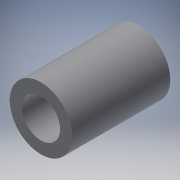
# Autodesk Inventor part: newRollerBearing
Saved by Autodesk Inventor 2019 (Build 230136000, 136)
## iProperties
Created: 2021-11-20
Part Number: newRollerBearing
Material: Generic
Document SubType Name: Modeling
Designer: Ian
Density: 1 g/cm^3
Appearance: Default
Author: Ian
Autodesk Inventor part; units mm, degrees
ref_plane "YZ Plane" through (0, 0, 0) normal (1, 0, 0) x (0, 1, 0)
ref_plane "XZ Plane" through (0, 0, 0) normal (0, 1, 0) x (-1, 0, 0)
ref_plane "XY Plane" through (0, 0, 0) normal (0, 0, 1) x (1, 0, 0)
sketch "Sketch1" plane through (0, 0, 0) normal (0, 0, 1) x (1, 0, 0)
  circle A0 centre (0, -1.9394) radius 2 construction
  circle A1 centre (0, -1.9394) radius 2.15
  circle A2 centre (0, -1.9394) radius 4
  point P0 (0, 0)
  dimension "d0" = 4
  dimension "d1" = 0.15
  dimension "d2" = 8
  constraints: 2 centre point, 1 coincident
  measures "d0" diameter of A0
  measures "d1" radial gap between concentric circles of A0 A1
  measures "d2" diameter of A2
extrude "Extrusion1" add sketch "Sketch1" along normal blind 11
sketch "Sketch2" plane through (0, 0, 0) normal (1, 0, 0) x (0, 1, 0)
  line L0 (2.0606, 0) -> (2.0606, 11) construction
  line L1 (-11.0374, 8.4) -> (-11.0374, 8.56) construction
  line L2 (-11.6374, 9.04) -> (-11.6374, 8.88) construction
  line L3 (-11.0374, 9.36) -> (-11.6374, 9.04) construction
  line L4 (-11.6374, 8.88) -> (-11.0374, 8.56) construction
  line L5 (-11.0374, 8.4) -> (-11.6374, 8.08) construction
  line L6 (-11.6374, 8.08) -> (-11.6374, 7.92) construction
  line L7 (-11.6374, 7.92) -> (-11.0374, 7.6) construction
  line L8 (-11.6374, 8.88) -> (2.0606, 8.88) construction
  line L9 (2.0606, 8.88) -> (1.4606, 8.56)
  line L10 (1.4606, 8.56) -> (1.4606, 8.4)
  line L11 (1.4606, 8.4) -> (2.0606, 8.08)
  line L12 (2.0606, 8.08) -> (2.0606, 7.92)
  line L13 (2.0606, 7.12) -> (2.0606, 6.96)
  line L14 (1.4606, 7.44) -> (2.0606, 7.12)
  line L15 (1.4606, 7.6) -> (1.4606, 7.44)
  line L16 (2.0606, 7.92) -> (1.4606, 7.6)
  line L17 (2.0606, 6.16) -> (2.0606, 6)
  line L18 (1.4606, 6.48) -> (2.0606, 6.16)
  line L19 (1.4606, 6.64) -> (1.4606, 6.48)
  line L20 (2.0606, 6.96) -> (1.4606, 6.64)
  line L21 (2.0606, 5.2) -> (2.0606, 5.04)
  line L22 (1.4606, 5.52) -> (2.0606, 5.2)
  line L23 (1.4606, 5.68) -> (1.4606, 5.52)
  line L24 (2.0606, 6) -> (1.4606, 5.68)
  line L25 (2.0606, 4.24) -> (2.0606, 4.08)
  line L26 (1.4606, 4.56) -> (2.0606, 4.24)
  line L27 (1.4606, 4.72) -> (1.4606, 4.56)
  line L28 (2.0606, 5.04) -> (1.4606, 4.72)
  line L29 (2.0606, 3.28) -> (2.0606, 3.12)
  line L30 (1.4606, 3.6) -> (2.0606, 3.28)
  line L31 (1.4606, 3.76) -> (1.4606, 3.6)
  line L32 (2.0606, 4.08) -> (1.4606, 3.76)
  line L33 (2.0606, 2.32) -> (2.0606, 2.16)
  line L34 (1.4606, 2.64) -> (2.0606, 2.32)
  line L35 (1.4606, 2.8) -> (1.4606, 2.64)
  line L36 (2.0606, 3.12) -> (1.4606, 2.8)
  line L37 (2.0606, 8.88) -> (2.0606, 8.08)
  line L38 (2.0606, 7.92) -> (2.0606, 7.12)
  line L39 (2.0606, 6.96) -> (2.0606, 6.16)
  line L40 (2.0606, 6) -> (2.0606, 5.2)
  line L41 (2.0606, 5.04) -> (2.0606, 4.24)
  line L42 (2.0606, 4.08) -> (2.0606, 3.28)
  line L43 (2.0606, 3.12) -> (2.0606, 2.32)
  line L44 (-1.9394, 10.1386) -> (-1.9394, 4.0681) construction
  line L45 (0.2106, 0) -> (0.2106, 11) construction
  line L46 (-4.0894, 0) -> (-4.0894, 11) construction
  point P0 (0, 0)
  dimension "d5" = 0.16
  dimension "d6" = 0.16
  dimension "d7" = 0.8
  dimension "d8" = 0.6
  dimension "d9" = 0.6
  dimension "d10" = 0.8
  dimension "d13" = 0.96
  dimension "d18" = 2.15
  dimension "d19" = 2.15
  constraints: 88 end point, 7 collinear, 6 vertical, 3 point on line, 1 equal length, 1 horizontal, 66 other
  measures "d5" distance of L9.end L10.end
  measures "d6" distance of L11.end L12.end
  measures "d7" distance of L11.end L8.end
  measures "d8" distance between parallel lines of L0 L10
  measures "d9" distance between parallel lines of L2 L1
  measures "d10" distance of L1.end L3.start
  measures "d13" distance of L11.end L13.start
  measures "d18" distance between parallel lines of L45 L44
  measures "d19" distance between parallel lines of L46 L44
revolve "Revolution1" cut sketch "Sketch2" angle 360 about axis through (0, -1.9394, 10.1386) along (0, 0, -1)
equation "\"d18\" = d19"
body "Solid1"
